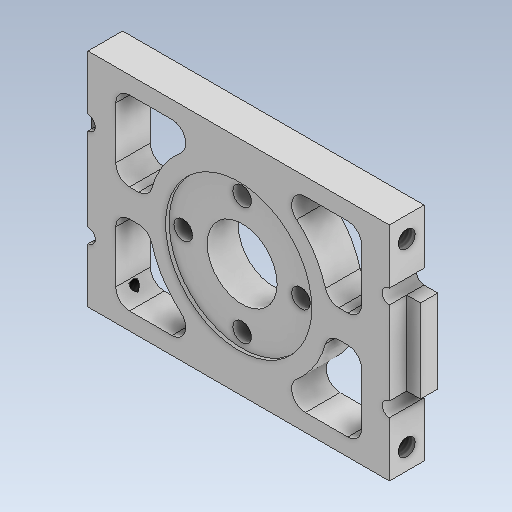
# Autodesk Inventor part: Shoulder_vertical_frame_01
Saved by Autodesk Inventor 2020.4 (Build 244396000, 396)
## iProperties
Created: 2021-09-24
Part Number: Shoulder_vertical_frame_01
Material: 一般
Document SubType Name: Modeling
Designer: Masato
Density: 1 g/cm^3
Appearance: 既定
Mass: 4.64191 g
Surface Area: 39.6043 cm^2
Volume: 4.64191 cm^3
Author: Masato Kubotera
Autodesk Inventor part; units mm, degrees
ref_plane "YZ Plane" through (0, 0, 0) normal (1, 0, 0) x (0, 1, 0)
ref_plane "XZ Plane" through (0, 0, 0) normal (0, 1, 0) x (-1, 0, 0)
ref_plane "XY Plane" through (0, 0, 0) normal (0, 0, 1) x (1, 0, 0)
sketch "スケッチ1" plane through (0, 0, 0) normal (0, 0, 1) x (1, 0, 0)
  line L0 (-21.75, 16) -> (21.75, 16)
  line L1 (21.75, -16) -> (-21.75, -16)
  line L2 (-21.75, 16) -> (21.75, -16) construction
  line L3 (21.75, 16) -> (-21.75, -16) construction
  circle A0 centre (0, 0) radius 10.5 construction
  line L4 (0, 16) -> (0, -16) construction
  circle A1 centre (0, 8.5) radius 1.35
  circle A2 centre (-8.5, 0) radius 1.35
  circle A3 centre (0, -8.5) radius 1.35
  circle A4 centre (8.5, 0) radius 1.35
  line L5 (-21.75, 6) -> (-23.75, 6)
  line L6 (-23.75, 6) -> (-23.75, -6)
  arc A5 (-21.75, 6) -> (-21.75, 8.1) centre (-21.75, 7.05) ccw
  line L7 (-21.75, 8.1) -> (-21.75, 16)
  line L8 (-23.75, 0) -> (23.75, 0) construction
  line L9 (-21.75, -6) -> (-23.75, -6)
  arc A6 (-21.75, -8.1) -> (-21.75, -6) centre (-21.75, -7.05) ccw
  line L10 (-21.75, -8.1) -> (-21.75, -16)
  line L11 (23.75, 6) -> (23.75, -6)
  arc A7 (21.75, 8.1) -> (21.75, 6) centre (21.75, 7.05) ccw
  line L12 (21.75, 8.1) -> (21.75, 16)
  line L13 (21.75, -6) -> (23.75, -6)
  line L14 (21.75, -8.1) -> (21.75, -16)
  arc A8 (21.75, -6) -> (21.75, -8.1) centre (21.75, -7.05) ccw
  line L15 (21.75, 6) -> (23.75, 6)
  line L16 (-21.75, 14.55) -> (-15.75, 14.55) construction
  line L17 (-15.75, 14.55) -> (-15.75, 11.45) construction
  line L18 (-15.75, 11.45) -> (-21.75, 11.45) construction
  line L19 (-15.75, 13) -> (-21.75, 13) construction
  arc A9 (-2, 12.8452) -> (-12.8452, 2) centre (0, 0) ccw
  circle A10 centre (0, 0) radius 5.05
  line L20 (-12.8452, 2) -> (-17.75, 2)
  line L21 (-17.75, 2) -> (-17.75, 13.5)
  line L22 (-17.75, 13.5) -> (-2, 13.5)
  line L23 (-2, 13.5) -> (-2, 12.8452)
  arc A11 (-12.8452, -2) -> (-2, -12.8452) centre (0, 0) ccw
  line L24 (-12.8452, -2) -> (-17.75, -2)
  line L25 (-17.75, -2) -> (-17.75, -13.5)
  line L26 (-17.75, -13.5) -> (-2, -13.5)
  line L27 (-2, -13.5) -> (-2, -12.8452)
  arc A12 (12.8452, 2) -> (2, 12.8452) centre (0, 0) ccw
  line L28 (12.8452, 2) -> (17.75, 2)
  line L29 (17.75, 2) -> (17.75, 13.5)
  line L30 (17.75, 13.5) -> (2, 13.5)
  line L31 (2, 13.5) -> (2, 12.8452)
  line L32 (12.8452, -2) -> (17.75, -2)
  arc A13 (2, -12.8452) -> (12.8452, -2) centre (0, 0) ccw
  line L33 (17.75, -13.5) -> (2, -13.5)
  line L34 (17.75, -2) -> (17.75, -13.5)
  line L35 (2, -13.5) -> (2, -12.8452)
  circle A14 centre (0, 0) radius 10.55
  circle A15 centre (0, 0) radius 5 construction
  line L36 (-21.75, 6) -> (-21.75, -6)
  line L37 (21.75, 6) -> (21.75, -6)
  point P0 (0, 0)
  dimension "d0" = 21
  dimension "d1" = 2.7
  dimension "d2" = 8.5
  dimension "d5" = 360
  dimension "d7" = 43.5
  dimension "d8" = 32
  dimension "d10" = 10
  dimension "d11" = 1.05
  dimension "d12" = 2
  dimension "d13" = 3.1
  dimension "d14" = 6
  dimension "d15" = 7
  dimension "d17" = 4
  dimension "d18" = 2.5
  dimension "d19" = 2.5
  dimension "d20" = 4
  dimension "d21" = 4
  dimension "d22" = 10
  dimension "d23" = 0.05
  dimension "d24" = 0.05
  constraints: 76 end point, 27 symmetric about line, 17 point on circle, 16 centre point, 9 midpoint, 8 perpendicular, 8 point on line, 5 coincident, 5 horizontal, 2 parallel, 1 tangent, 1 vertical, 15 other
  measures "d0" diameter of A0
  measures "d1" diameter of A1
  measures "d2" distance of point (0, 0) A1.centre
  measures "d7" distance of L0.end L0.start
  measures "d8" distance of L1.end L0.start
  measures "d10" distance of L0.start L5.start
  measures "d11" radius of A5
  measures "d12" distance of L5.start L5.end
  measures "d13" distance of L17.end L16.end
  measures "d14" distance of L16.start L16.end
  measures "d15" vertical distance of L5.end L19.end
  measures "d17" horizontal distance of L0.start L21.end
  measures "d18" vertical distance of L0.start L21.end
  measures "d19" radial gap between concentric circles of A9 A0
  measures "d20" distance of L22.end L30.end
  measures "d21" distance of L24.end L20.end
  measures "d22" diameter of A15
  measures "d23" radial gap between concentric circles of A15 A10
  measures "d24" radial gap between concentric circles of A14 A0
extrude "押し出し1" add sketch "スケッチ1" along normal blind 5 contours L0 L12 A7 L37 A8 L14 L1 L10 A6 L36 A5 L7
extrude "押し出し2" add sketch "スケッチ1" along normal blind 4.5 contours A14
extrude "押し出し3" add sketch "スケッチ1" along normal blind 2.5 contours L36 L9 L6 L5 | L15 L11 L13 L37
fillet "フィレット1" radius 2 20 edges at (-17.75, 13.5, 2.5) (-2, 13.5, 2.5) (-2, 12.8452, 2.5) (-12.8452, 2, 2.5) (-17.75, 2, 2.5) (-17.75, -2, 2.5) (-12.8452, -2, 2.5) (-17.75, -13.5, 2.5) (-2, -13.5, 2.5) (-2, -12.8452, 2.5) (2, -12.8452, 2.5) (2, -13.5, 2.5) (12.8452, -2, 2.5) (17.75, -2, 2.5) (17.75, -13.5, 2.5) (17.75, 2, 2.5) (12.8452, 2, 2.5) (2, 13.5, 2.5) (2, 12.8452, 2.5) (17.75, 13.5, 2.5)
sketch "スケッチ2" plane through (-21.75, 8.1, 0) normal (-1, 0, 0) x (0, 0, 1)
  line L0 (0, 7.9) -> (0, 0) projected
  line L1 (0, -16.2) -> (0, -24.1) projected
  line L2 (2.5, -2.1) -> (5, -2.1) projected
  line L3 (2.5, -14.1) -> (5, -14.1) projected
  point P0 (0, -8.1)
  point P1 (2.5, 4.9)
  point P2 (2.5, -21.1)
  point P3 (0, -2.1)
  point P4 (0, -14.1)
  dimension "d30" = 2.5
  dimension "d32" = 2.5
  dimension "d50" = 7
  dimension "d51" = 7
  measures "d30" distance from line of L0 point (2.5, 4.9)
  measures "d32" distance from line of L1 point (2.5, -21.1)
  measures "d50" distance from line of point (2.5, 4.9) L2
  measures "d51" distance from line of point (2.5, -21.1) L3
hole "穴1" at (-21.75, 13, 2.5) at (-21.75, -13, 2.5) direction (1, 0, 0) diameter 2.459 depth 4 tip angle 118 thread size "M3x0.5" class "6H" standard "ISO Metric profile"
sketch "スケッチ3" plane through (21.75, 8.1, 0) normal (1, 0, 0) x (0, 0, -1)
  circle A0 centre (-2.5, 4.9) radius 1.2295 projected
  circle A1 centre (-2.5, -21.1) radius 1.2295 projected
  point P0 (0, -8.1)
  constraints: 2 coincident
hole "穴2" at (21.75, 13, 2.5) at (21.75, -13, 2.5) direction (-1, 0, 0) diameter 2.459 depth 4 tip angle 118 thread size "M3x0.5" class "6H" standard "ISO Metric profile"
equation "\"d19\" = d18"
equation "\"d24\" = d23"
equation "\"d32\" = d30"
equation "\"d50\" = d15"
equation "\"d51\" = d50"
